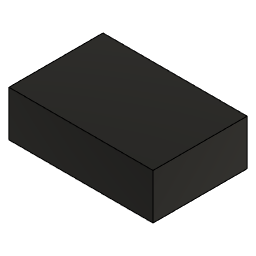
Pi casing v4 (Autodesk Fusion 360 design; units mm, degrees)
Autodesk Fusion 360 part; units mm, degrees
sketch "Sketch1" plane through (0, 0, 0) normal (0, 0, 1) x (1, 0, 0)
  line L0 (47.5, -31) -> (-47.5, -31)
  line L1 (-47.5, -31) -> (-47.5, 31)
  line L2 (-47.5, 31) -> (47.5, 31)
  line L3 (47.5, 31) -> (47.5, -31)
  line L4 (47.5, -31) -> (-47.5, 31) construction
  line L5 (-47.5, -31) -> (47.5, 31) construction
  dimension "d1" = 95
  dimension "d2" = 62
  constraint horizontal L0
  constraint perpendicular L0 L1
  constraint parallel L0 L2
  constraint parallel L1 L3
  constraint coincident L4 origin
  constraint coincident L5 origin
  measures "d1" distance of L1.end L2.end
  measures "d2" distance of L0.end L1.end
surface "Extrude1" add extruded along (0, 0, 1) between 0 and 30 profiles "Sketch1" section 1 makes body 1
surface "SurfacePatch1" add patch along 4 edges at (47.5, 0, 30) (0, 31, 30) (-47.5, 0, 30) (0, -31, 30) separate body on bodies 1 makes body 2
surface "SurfacePatch2" add patch along 4 edges at (0, 31, 0) (47.5, 0, 0) (0, -31, 0) (-47.5, 0, 0) separate body on bodies 1 makes body 3
stitch "SurfaceStitch1" surfaces 3 2 1 tolerance 0.1 makes body 4
